Autodesk Inventor part; units mm, degrees
(part 3 of 4)
  arc A461 (22.2112, 13.7256) -> (22.0661, 14.076) centre (4.2393, 6.4866) ccw
  arc A462 (22.0661, 14.076) -> (22.3098, 14.2726) centre (18.8793, 18.2757) ccw
  arc A463 (22.3098, 14.2726) -> (22.601, 14.538) centre (18.1407, 19.1385) ccw
  arc A464 (22.601, 14.538) -> (22.939, 14.8874) centre (17.3199, 19.9858) ccw
  arc A465 (22.939, 14.8874) -> (22.7717, 15.2501) centre (4.2393, 6.4866) ccw
  arc A466 (22.7717, 15.2501) -> (22.2866, 15.22) centre (22.9993, 7.6662) ccw
  arc A467 (22.2866, 15.22) -> (21.8956, 15.171) centre (22.8881, 8.8406) ccw
  arc A468 (21.8956, 15.171) -> (21.5878, 15.1133) centre (22.7117, 9.9626) ccw
  arc A469 (21.5878, 15.1133) -> (21.4156, 15.4512) centre (4.2393, 6.4866) ccw
  arc A470 (21.4156, 15.4512) -> (21.6432, 15.6664) centre (17.9092, 19.388) ccw
  arc A471 (21.6432, 15.6664) -> (21.9127, 15.9538) centre (17.1052, 20.1902) ccw
  arc A472 (21.9127, 15.9538) -> (22.2222, 16.3286) centre (16.2205, 20.9705) ccw
  arc A473 (22.2222, 16.3286) -> (22.027, 16.6771) centre (4.2393, 6.4866) ccw
  arc A474 (22.027, 16.6771) -> (21.5457, 16.609) centre (22.8489, 9.1345) ccw
  arc A475 (21.5457, 16.609) -> (21.1598, 16.5295) centre (22.646, 10.2965) ccw
  arc A476 (21.1598, 16.5295) -> (20.8575, 16.4479) centre (22.3821, 11.4012) ccw
  arc A477 (20.8575, 16.4479) -> (20.6593, 16.7712) centre (4.2393, 6.4866) ccw
  arc A478 (20.6593, 16.7712) -> (20.8693, 17.0036) centre (16.8549, 20.4208) ccw
  arc A479 (20.8693, 17.0036) -> (21.1154, 17.3113) centre (15.9904, 21.1574) ccw
  arc A480 (21.1154, 17.3113) -> (21.3946, 17.7092) centre (15.0472, 21.8658) ccw
  arc A481 (21.3946, 17.7092) -> (21.1727, 18.0413) centre (4.2393, 6.4866) ccw
  arc A482 (21.1727, 18.0413) -> (20.6982, 17.9357) centre (22.5838, 10.5864) ccw
  arc A483 (20.6982, 17.9357) -> (20.3197, 17.8261) centre (22.2903, 11.7289) ccw
  arc A484 (20.3197, 17.8261) -> (20.0247, 17.721) centre (21.9406, 12.8095) ccw
  arc A485 (20.0247, 17.721) -> (19.8018, 18.0278) centre (4.2393, 6.4866) ccw
  arc A486 (19.8018, 18.0278) -> (19.9929, 18.2759) centre (15.7227, 21.3676) ccw
  arc A487 (19.9929, 18.2759) -> (20.2141, 18.602) centre (14.8031, 22.0342) ccw
  arc A488 (20.2141, 18.602) -> (20.4612, 19.0206) centre (13.8072, 22.6664) ccw
  arc A489 (20.4612, 19.0206) -> (20.2139, 19.3343) centre (4.2393, 6.4866) ccw
  arc A490 (20.2139, 19.3343) -> (19.7492, 19.1917) centre (22.2056, 12.0131) ccw
  arc A491 (19.7492, 19.1917) -> (19.3805, 19.0528) centre (21.8234, 13.129) ccw
  arc A492 (19.3805, 19.0528) -> (19.0946, 18.9249) centre (21.3899, 14.1788) ccw
  arc A493 (19.0946, 18.9249) -> (18.8483, 19.2133) centre (4.2393, 6.4866) ccw
  arc A494 (18.8483, 19.2133) -> (19.0194, 19.4756) centre (14.5198, 22.2227) ccw
  arc A495 (19.0194, 19.4756) -> (19.2143, 19.818) centre (13.5507, 22.8151) ccw
  arc A496 (19.2143, 19.818) -> (19.4278, 20.2547) centre (12.5083, 23.3672) ccw
  arc A497 (19.4278, 20.2547) -> (19.1566, 20.548) centre (4.2393, 6.4866) ccw
  arc A498 (19.1566, 20.548) -> (18.7045, 20.3695) centre (21.7166, 13.4056) ccw
  arc A499 (18.7045, 20.3695) -> (18.3479, 20.202) centre (21.248, 14.4882) ccw
  arc A500 (18.3479, 20.202) -> (18.0729, 20.0521) centre (20.7335, 15.5007) ccw
  arc A501 (18.0729, 20.0521) -> (17.8048, 20.3202) centre (4.2393, 6.4866) ccw
  arc A502 (17.8048, 20.3202) -> (17.9547, 20.5952) centre (13.2534, 22.9808) ccw
  arc A503 (17.9547, 20.5952) -> (18.1221, 20.9518) centre (12.2409, 23.4953) ccw
  arc A504 (18.1221, 20.9518) -> (18.3007, 21.4039) centre (11.1583, 23.964) ccw
  arc A505 (18.3007, 21.4039) -> (18.0074, 21.6751) centre (4.2393, 6.4866) ccw
  arc A506 (18.0074, 21.6751) -> (17.5707, 21.4616) centre (21.1199, 14.7556) ccw
  arc A507 (17.5707, 21.4616) -> (17.2283, 21.2667) centre (20.5678, 15.798) ccw
  arc A508 (17.2283, 21.2667) -> (16.966, 21.0956) centre (19.9754, 16.7671) ccw
  arc A509 (16.966, 21.0956) -> (16.6776, 21.3419) centre (4.2393, 6.4866) ccw
  arc A510 (16.6776, 21.3419) -> (16.8055, 21.6278) centre (11.9315, 23.6372) ccw
  arc A511 (16.8055, 21.6278) -> (16.9444, 21.9965) centre (10.8817, 24.0707) ccw
  arc A512 (16.9444, 21.9965) -> (17.087, 22.4612) centre (9.7657, 24.4529) ccw
  arc A513 (17.087, 22.4612) -> (16.7733, 22.7085) centre (4.2393, 6.4866) ccw
  arc A514 (16.7733, 22.7085) -> (16.3547, 22.4614) centre (20.4191, 16.0545) ccw
  arc A515 (16.3547, 22.4614) -> (16.0286, 22.2402) centre (19.7869, 17.0504) ccw
  arc A516 (16.0286, 22.2402) -> (15.7805, 22.0491) centre (19.1203, 17.97) ccw
  arc A517 (15.7805, 22.0491) -> (15.4737, 22.272) centre (4.2393, 6.4866) ccw
  arc A518 (15.4737, 22.272) -> (15.5788, 22.567) centre (10.5622, 24.1879) ccw
  arc A519 (15.5788, 22.567) -> (15.6884, 22.9455) centre (9.4816, 24.5376) ccw
  arc A520 (15.6884, 22.9455) -> (15.794, 23.42) centre (8.3391, 24.8311) ccw
  arc A521 (15.794, 23.42) -> (15.4619, 23.6419) centre (4.2393, 6.4866) ccw
  arc A522 (15.4619, 23.6419) -> (15.064, 23.3627) centre (19.6185, 17.2945) ccw
  arc A523 (15.064, 23.3627) -> (14.7563, 23.1166) centre (18.9101, 18.2377) ccw
  arc A524 (14.7563, 23.1166) -> (14.5239, 22.9067) centre (18.1735, 19.1022) ccw
  arc A525 (14.5239, 22.9067) -> (14.2006, 23.1048) centre (4.2393, 6.4866) ccw
  arc A526 (14.2006, 23.1048) -> (14.2822, 23.4072) centre (9.1539, 24.6294) ccw
  arc A527 (14.2822, 23.4072) -> (14.3617, 23.793) centre (8.0492, 24.8933) ccw
  arc A528 (14.3617, 23.793) -> (14.4298, 24.2743) centre (6.8872, 25.0963) ccw
  arc A529 (14.4298, 24.2743) -> (14.0813, 24.4695) centre (4.2393, 6.4866) ccw
  arc A530 (14.0813, 24.4695) -> (13.7065, 24.16) centre (18.7231, 18.4678) ccw
  arc A531 (13.7065, 24.16) -> (13.4191, 23.8905) centre (17.9429, 19.3525) ccw
  arc A532 (13.4191, 23.8905) -> (13.2039, 23.663) centre (17.1407, 20.1566) ccw
  arc A533 (13.2039, 23.663) -> (12.866, 23.8351) centre (4.2393, 6.4866) ccw
  arc A534 (12.866, 23.8351) -> (12.9236, 24.143) centre (7.7153, 24.9591) ccw
  arc A535 (12.9236, 24.143) -> (12.9727, 24.5339) centre (6.5933, 25.1355) ccw
  arc A536 (12.9727, 24.5339) -> (13.0028, 25.0191) centre (5.4189, 25.2466) ccw
  arc A537 (13.0028, 25.0191) -> (12.64, 25.1863) centre (4.2393, 6.4866) ccw
  arc A538 (12.64, 25.1863) -> (12.2907, 24.8483) centre (17.7385, 19.5672) ccw
  arc A539 (12.2907, 24.8483) -> (12.0253, 24.5571) centre (16.8912, 20.388) ccw
  arc A540 (12.0253, 24.5571) -> (11.8286, 24.3134) centre (16.0284, 21.1266) ccw
  arc A541 (11.8286, 24.3134) -> (11.4783, 24.4585) centre (4.2393, 6.4866) ccw
  arc A542 (11.4783, 24.4585) -> (11.5116, 24.7699) centre (6.2552, 25.1748) ccw
  arc A543 (11.5116, 24.7699) -> (11.5298, 25.1635) centre (5.1228, 25.2627) ccw
  arc A544 (11.5298, 25.1635) -> (11.5218, 25.6495) centre (3.9434, 25.2814) ccw
  arc A545 (11.5218, 25.6495) -> (11.147, 25.7878) centre (4.2393, 6.4866) ccw
  arc A546 (11.147, 25.7878) -> (10.8252, 25.4234) centre (16.6706, 20.5861) ccw
  arc A547 (10.8252, 25.4234) -> (10.5835, 25.1123) centre (15.7615, 21.3378) ccw
  arc A548 (10.5835, 25.1123) -> (10.4066, 24.8539) centre (14.8434, 22.0065) ccw
  arc A549 (10.4066, 24.8539) -> (10.0459, 24.9711) centre (4.2393, 6.4866) ccw
  arc A550 (10.0459, 24.9711) -> (10.0547, 25.2841) centre (4.7827, 25.2754) ccw
  arc A551 (10.0547, 25.2841) -> (10.0419, 25.6779) centre (3.647, 25.2741) ccw
  arc A552 (10.0419, 25.6779) -> (9.9958, 26.1618) centre (2.4697, 25.2002) ccw
  arc A553 (9.9958, 26.1618) -> (9.6113, 26.2702) centre (4.2393, 6.4866) ccw
  arc A554 (9.6113, 26.2702) -> (9.3192, 25.8817) centre (15.526, 21.5179) ccw
  arc A555 (9.3192, 25.8817) -> (9.1026, 25.5526) centre (14.5608, 22.1961) ccw
  arc A556 (9.1026, 25.5526) -> (8.9465, 25.2811) centre (13.5931, 22.7906) ccw
  arc A557 (8.9465, 25.2811) -> (8.5777, 25.3697) centre (4.2393, 6.4866) ccw
  arc A558 (8.5777, 25.3697) -> (8.5619, 25.6824) centre (3.3069, 25.2601) ccw
  arc A559 (8.5619, 25.6824) -> (8.5183, 26.074) centre (2.1747, 25.1697) ccw
  arc A560 (8.5183, 26.074) -> (8.4344, 26.5528) centre (1.0069, 25.0037) ccw
  arc A561 (8.4344, 26.5528) -> (8.0426, 26.6307) centre (4.2393, 6.4866) ccw
  arc A562 (8.0426, 26.6307) -> (7.7818, 26.2205) centre (14.3119, 22.3571) ccw
  arc A563 (7.7818, 26.2205) -> (7.5917, 25.8754) centre (13.2964, 22.9575) ccw
  arc A564 (7.5917, 25.8754) -> (7.4574, 25.5925) centre (12.285, 23.4742) ccw
  arc A565 (7.4574, 25.5925) -> (7.0828, 25.6518) centre (4.2393, 6.4866) ccw
  arc A566 (7.0828, 25.6518) -> (7.0425, 25.9624) centre (1.8368, 25.1291) ccw
  arc A567 (7.0425, 25.9624) -> (6.9683, 26.3493) centre (0.7152, 24.9501) ccw
  arc A568 (6.9683, 26.3493) -> (6.8471, 26.8201) centre (-0.436, 24.693) ccw
  arc A569 (6.8471, 26.8201) -> (6.4504, 26.867) centre (4.2393, 6.4866) ccw
  arc A570 (6.4504, 26.867) -> (6.2226, 26.4376) centre (13.0356, 23.0985) ccw
  arc A571 (6.2226, 26.4376) -> (6.0601, 26.0787) centre (11.9762, 23.6173) ccw
  arc A572 (6.0601, 26.0787) -> (5.9484, 25.7861) centre (10.9274, 24.0531) ccw
  arc A573 (5.9484, 25.7861) -> (5.5703, 25.8158) centre (4.2393, 6.4866) ccw
  arc A574 (5.5703, 25.8158) -> (5.5058, 26.1223) centre (0.3816, 24.8831) ccw
  arc A575 (5.5058, 26.1223) -> (5.4015, 26.5022) centre (-0.7225, 24.6167) ccw
  arc A576 (5.4015, 26.5022) -> (5.2437, 26.962) centre (-1.85, 24.27) ccw
  arc A577 (5.2437, 26.962) -> (4.8445, 26.9777) centre (4.2393, 6.4866) ccw
  arc A578 (4.8445, 26.9777) -> (4.6511, 26.5317) centre (11.7052, 23.7374) ccw
  arc A579 (4.6511, 26.5317) -> (4.5173, 26.1611) centre (10.6083, 24.1715) ccw
  arc A580 (4.5173, 26.1611) -> (4.4289, 25.8607) centre (9.5285, 24.5237) ccw
  arc A581 (4.4289, 25.8607) -> (4.0497, 25.8607) centre (4.2393, 6.4866) ccw
  arc A582 (4.0497, 25.8607) -> (3.9613, 26.1611) centre (-1.0499, 24.5237) ccw
  arc A583 (3.9613, 26.1611) -> (3.8275, 26.5317) centre (-2.1297, 24.1715) ccw
  arc A584 (3.8275, 26.5317) -> (3.6341, 26.9777) centre (-3.2265, 23.7374) ccw
  arc A585 (3.6341, 26.9777) -> (3.2349, 26.962) centre (4.2393, 6.4866) ccw
  arc A586 (3.2349, 26.962) -> (3.0771, 26.5022) centre (10.3287, 24.27) ccw
  arc A587 (3.0771, 26.5022) -> (2.9728, 26.1223) centre (9.2011, 24.6167) ccw
  arc A588 (2.9728, 26.1223) -> (2.9083, 25.8158) centre (8.097, 24.8831) ccw
  arc A589 (2.9083, 25.8158) -> (2.5302, 25.7861) centre (4.2393, 6.4866) ccw
  arc A590 (2.5302, 25.7861) -> (2.4185, 26.0787) centre (-2.4488, 24.0531) ccw
  arc A591 (2.4185, 26.0787) -> (2.2561, 26.4376) centre (-3.4976, 23.6173) ccw
  arc A592 (2.2561, 26.4376) -> (2.0283, 26.867) centre (-4.557, 23.0985) ccw
  arc A593 (2.0283, 26.867) -> (1.6316, 26.8201) centre (4.2393, 6.4866) ccw
  arc A594 (1.6316, 26.8201) -> (1.5103, 26.3493) centre (8.9146, 24.693) ccw
  arc A595 (1.5103, 26.3493) -> (1.4361, 25.9624) centre (7.7634, 24.9501) ccw
  arc A596 (1.4361, 25.9624) -> (1.3958, 25.6518) centre (6.6418, 25.1291) ccw
  arc A597 (1.3958, 25.6518) -> (1.0212, 25.5925) centre (4.2393, 6.4866) ccw
  arc A598 (1.0212, 25.5925) -> (0.887, 25.8754) centre (-3.8064, 23.4742) ccw
  arc A599 (0.887, 25.8754) -> (0.6968, 26.2205) centre (-4.8178, 22.9575) ccw
  arc A600 (0.6968, 26.2205) -> (0.436, 26.6307) centre (-5.8332, 22.3571) ccw
  arc A601 (0.436, 26.6307) -> (0.0443, 26.5528) centre (4.2393, 6.4866) ccw
  arc A602 (0.0443, 26.5528) -> (-0.0397, 26.074) centre (7.4718, 25.0037) ccw
  arc A603 (-0.0397, 26.074) -> (-0.0833, 25.6824) centre (6.3039, 25.1697) ccw
  arc A604 (-0.0833, 25.6824) -> (-0.0991, 25.3697) centre (5.1717, 25.2601) ccw
  arc A605 (-0.0991, 25.3697) -> (-0.4679, 25.2811) centre (4.2393, 6.4866) ccw
  arc A606 (-0.4679, 25.2811) -> (-0.6239, 25.5526) centre (-5.1144, 22.7906) ccw
  arc A607 (-0.6239, 25.5526) -> (-0.8405, 25.8817) centre (-6.0822, 22.1961) ccw
  arc A608 (-0.8405, 25.8817) -> (-1.1327, 26.2702) centre (-7.0474, 21.5179) ccw
  arc A609 (-1.1327, 26.2702) -> (-1.5172, 26.1618) centre (4.2393, 6.4866) ccw
  arc A610 (-1.5172, 26.1618) -> (-1.5633, 25.6779) centre (6.009, 25.2002) ccw
  arc A611 (-1.5633, 25.6779) -> (-1.576, 25.2841) centre (4.8317, 25.2741) ccw
  arc A612 (-1.576, 25.2841) -> (-1.5673, 24.9711) centre (3.6959, 25.2754) ccw
  arc A613 (-1.5673, 24.9711) -> (-1.928, 24.8539) centre (4.2393, 6.4866) ccw
  arc A614 (-1.928, 24.8539) -> (-2.1048, 25.1123) centre (-6.3648, 22.0065) ccw
  arc A615 (-2.1048, 25.1123) -> (-2.3466, 25.4234) centre (-7.2829, 21.3378) ccw
  arc A616 (-2.3466, 25.4234) -> (-2.6684, 25.7878) centre (-8.1919, 20.5861) ccw
  arc A617 (-2.6684, 25.7878) -> (-3.0431, 25.6495) centre (4.2393, 6.4866) ccw
  arc A618 (-3.0431, 25.6495) -> (-3.0512, 25.1635) centre (4.5353, 25.2814) ccw
  arc A619 (-3.0512, 25.1635) -> (-3.033, 24.7699) centre (3.3558, 25.2627) ccw
  arc A620 (-3.033, 24.7699) -> (-2.9996, 24.4585) centre (2.2234, 25.1748) ccw
  arc A621 (-2.9996, 24.4585) -> (-3.35, 24.3134) centre (4.2393, 6.4866) ccw
  arc A622 (-3.35, 24.3134) -> (-3.5466, 24.5571) centre (-7.5498, 21.1266) ccw
  arc A623 (-3.5466, 24.5571) -> (-3.8121, 24.8483) centre (-8.4126, 20.388) ccw
  arc A624 (-3.8121, 24.8483) -> (-4.1614, 25.1863) centre (-9.2598, 19.5672) ccw
  arc A625 (-4.1614, 25.1863) -> (-4.5242, 25.0191) centre (4.2393, 6.4866) ccw
  arc A626 (-4.5242, 25.0191) -> (-4.4941, 24.5339) centre (3.0597, 25.2466) ccw
  arc A627 (-4.4941, 24.5339) -> (-4.445, 24.143) centre (1.8854, 25.1355) ccw
  arc A628 (-4.445, 24.143) -> (-4.3874, 23.8351) centre (0.7634, 24.9591) ccw
  arc A629 (-4.3874, 23.8351) -> (-4.7253, 23.663) centre (4.2393, 6.4866) ccw
  arc A630 (-4.7253, 23.663) -> (-4.9404, 23.8905) centre (-8.6621, 20.1566) ccw
  arc A631 (-4.9404, 23.8905) -> (-5.2279, 24.16) centre (-9.4643, 19.3525) ccw
  arc A632 (-5.2279, 24.16) -> (-5.6027, 24.4695) centre (-10.2445, 18.4678) ccw
  arc A633 (-5.6027, 24.4695) -> (-5.9512, 24.2743) centre (4.2393, 6.4866) ccw
  arc A634 (-5.9512, 24.2743) -> (-5.8831, 23.793) centre (1.5915, 25.0963) ccw
  arc A635 (-5.8831, 23.793) -> (-5.8036, 23.4072) centre (0.4294, 24.8933) ccw
  arc A636 (-5.8036, 23.4072) -> (-5.7219, 23.1048) centre (-0.6753, 24.6294) ccw
  arc A637 (-5.7219, 23.1048) -> (-6.0453, 22.9067) centre (4.2393, 6.4866) ccw
  arc A638 (-6.0453, 22.9067) -> (-6.2776, 23.1166) centre (-9.6948, 19.1022) ccw
  arc A639 (-6.2776, 23.1166) -> (-6.5853, 23.3627) centre (-10.4315, 18.2377) ccw
  circle A640 centre (4.2393, 6.4866) radius 2
  circle A641 centre (4.2393, 6.4866) radius 18.25
  point P0 (0, 0)
  dimension "d28" = 36.5
  constraints: 1 centre point, 1 coincident
  measures "d28" diameter of A641
extrude "押し出し8" cut sketch "スケッチ2" against normal blind 0.75 contours A641
sketch "スケッチ3" plane through (0, 0, 0) normal (0, 0, -1) x (-1, 0, 0)
  arc A0 (6.9833, 23.6419) -> (6.5853, 23.3627) centre (11.1399, 17.2945) ccw
  arc A1 (6.5853, 23.3627) -> (6.2776, 23.1166) centre (10.4315, 18.2377) ccw
  arc A2 (6.2776, 23.1166) -> (6.0453, 22.9067) centre (9.6948, 19.1022) ccw
  arc A3 (6.0453, 22.9067) -> (5.7219, 23.1048) centre (-4.2393, 6.4866) ccw
  arc A4 (5.7219, 23.1048) -> (5.8036, 23.4072) centre (0.6753, 24.6294) ccw
  arc A5 (5.8036, 23.4072) -> (5.8831, 23.793) centre (-0.4294, 24.8933) ccw
  arc A6 (5.8831, 23.793) -> (5.9512, 24.2743) centre (-1.5915, 25.0963) ccw
  arc A7 (5.9512, 24.2743) -> (5.6027, 24.4695) centre (-4.2393, 6.4866) ccw
  arc A8 (5.6027, 24.4695) -> (5.2279, 24.16) centre (10.2445, 18.4678) ccw
  arc A9 (5.2279, 24.16) -> (4.9404, 23.8905) centre (9.4643, 19.3525) ccw
  arc A10 (4.9404, 23.8905) -> (4.7253, 23.663) centre (8.6621, 20.1566) ccw
  arc A11 (4.7253, 23.663) -> (4.3874, 23.8351) centre (-4.2393, 6.4866) ccw
  arc A12 (4.3874, 23.8351) -> (4.445, 24.143) centre (-0.7634, 24.9591) ccw
  arc A13 (4.445, 24.143) -> (4.4941, 24.5339) centre (-1.8854, 25.1355) ccw
  arc A14 (4.4941, 24.5339) -> (4.5242, 25.0191) centre (-3.0597, 25.2466) ccw
  arc A15 (4.5242, 25.0191) -> (4.1614, 25.1863) centre (-4.2393, 6.4866) ccw
  arc A16 (4.1614, 25.1863) -> (3.8121, 24.8483) centre (9.2598, 19.5672) ccw
  arc A17 (3.8121, 24.8483) -> (3.5466, 24.5571) centre (8.4126, 20.388) ccw
  arc A18 (3.5466, 24.5571) -> (3.35, 24.3134) centre (7.5498, 21.1266) ccw
  arc A19 (3.35, 24.3134) -> (2.9996, 24.4585) centre (-4.2393, 6.4866) ccw
  arc A20 (2.9996, 24.4585) -> (3.033, 24.7699) centre (-2.2234, 25.1748) ccw
  arc A21 (3.033, 24.7699) -> (3.0512, 25.1635) centre (-3.3558, 25.2627) ccw
  arc A22 (3.0512, 25.1635) -> (3.0431, 25.6495) centre (-4.5353, 25.2814) ccw
  arc A23 (3.0431, 25.6495) -> (2.6684, 25.7878) centre (-4.2393, 6.4866) ccw
  arc A24 (2.6684, 25.7878) -> (2.3466, 25.4234) centre (8.1919, 20.5861) ccw
  arc A25 (2.3466, 25.4234) -> (2.1048, 25.1123) centre (7.2829, 21.3378) ccw
  arc A26 (2.1048, 25.1123) -> (1.928, 24.8539) centre (6.3648, 22.0065) ccw
  arc A27 (1.928, 24.8539) -> (1.5673, 24.9711) centre (-4.2393, 6.4866) ccw
  arc A28 (1.5673, 24.9711) -> (1.576, 25.2841) centre (-3.6959, 25.2754) ccw
  arc A29 (1.576, 25.2841) -> (1.5633, 25.6779) centre (-4.8317, 25.2741) ccw
  arc A30 (1.5633, 25.6779) -> (1.5172, 26.1618) centre (-6.009, 25.2002) ccw
  arc A31 (1.5172, 26.1618) -> (1.1327, 26.2702) centre (-4.2393, 6.4866) ccw
  arc A32 (1.1327, 26.2702) -> (0.8405, 25.8817) centre (7.0474, 21.5179) ccw
  arc A33 (0.8405, 25.8817) -> (0.6239, 25.5526) centre (6.0822, 22.1961) ccw
  arc A34 (0.6239, 25.5526) -> (0.4679, 25.2811) centre (5.1144, 22.7906) ccw
  arc A35 (0.4679, 25.2811) -> (0.0991, 25.3697) centre (-4.2393, 6.4866) ccw
  arc A36 (0.0991, 25.3697) -> (0.0833, 25.6824) centre (-5.1717, 25.2601) ccw
  arc A37 (0.0833, 25.6824) -> (0.0397, 26.074) centre (-6.3039, 25.1697) ccw
  arc A38 (0.0397, 26.074) -> (-0.0443, 26.5528) centre (-7.4718, 25.0037) ccw
  arc A39 (-0.0443, 26.5528) -> (-0.436, 26.6307) centre (-4.2393, 6.4866) ccw
  arc A40 (-0.436, 26.6307) -> (-0.6968, 26.2205) centre (5.8332, 22.3571) ccw
  arc A41 (-0.6968, 26.2205) -> (-0.887, 25.8754) centre (4.8178, 22.9575) ccw
  arc A42 (-0.887, 25.8754) -> (-1.0212, 25.5925) centre (3.8064, 23.4742) ccw
  arc A43 (-1.0212, 25.5925) -> (-1.3958, 25.6518) centre (-4.2393, 6.4866) ccw
  arc A44 (-1.3958, 25.6518) -> (-1.4361, 25.9624) centre (-6.6418, 25.1291) ccw
  arc A45 (-1.4361, 25.9624) -> (-1.5103, 26.3493) centre (-7.7634, 24.9501) ccw
  arc A46 (-1.5103, 26.3493) -> (-1.6316, 26.8201) centre (-8.9146, 24.693) ccw
  arc A47 (-1.6316, 26.8201) -> (-2.0283, 26.867) centre (-4.2393, 6.4866) ccw
  arc A48 (-2.0283, 26.867) -> (-2.2561, 26.4376) centre (4.557, 23.0985) ccw
  arc A49 (-2.2561, 26.4376) -> (-2.4185, 26.0787) centre (3.4976, 23.6173) ccw
  arc A50 (-2.4185, 26.0787) -> (-2.5302, 25.7861) centre (2.4488, 24.0531) ccw
  arc A51 (-2.5302, 25.7861) -> (-2.9083, 25.8158) centre (-4.2393, 6.4866) ccw
  arc A52 (-2.9083, 25.8158) -> (-2.9728, 26.1223) centre (-8.097, 24.8831) ccw
  arc A53 (-2.9728, 26.1223) -> (-3.0771, 26.5022) centre (-9.2011, 24.6167) ccw
  arc A54 (-3.0771, 26.5022) -> (-3.2349, 26.962) centre (-10.3287, 24.27) ccw
  arc A55 (-3.2349, 26.962) -> (-3.6341, 26.9777) centre (-4.2393, 6.4866) ccw
  arc A56 (-3.6341, 26.9777) -> (-3.8275, 26.5317) centre (3.2265, 23.7374) ccw
  arc A57 (-3.8275, 26.5317) -> (-3.9613, 26.1611) centre (2.1297, 24.1715) ccw
  arc A58 (-3.9613, 26.1611) -> (-4.0497, 25.8607) centre (1.0499, 24.5237) ccw
  arc A59 (-4.0497, 25.8607) -> (-4.4289, 25.8607) centre (-4.2393, 6.4866) ccw
  arc A60 (-4.4289, 25.8607) -> (-4.5173, 26.1611) centre (-9.5285, 24.5237) ccw
  arc A61 (-4.5173, 26.1611) -> (-4.6511, 26.5317) centre (-10.6083, 24.1715) ccw
  arc A62 (-4.6511, 26.5317) -> (-4.8445, 26.9777) centre (-11.7052, 23.7374) ccw
  arc A63 (-4.8445, 26.9777) -> (-5.2437, 26.962) centre (-4.2393, 6.4866) ccw
  arc A64 (-5.2437, 26.962) -> (-5.4015, 26.5022) centre (1.85, 24.27) ccw
  arc A65 (-5.4015, 26.5022) -> (-5.5058, 26.1223) centre (0.7225, 24.6167) ccw
  arc A66 (-5.5058, 26.1223) -> (-5.5703, 25.8158) centre (-0.3816, 24.8831) ccw
  arc A67 (-5.5703, 25.8158) -> (-5.9484, 25.7861) centre (-4.2393, 6.4866) ccw
  arc A68 (-5.9484, 25.7861) -> (-6.0601, 26.0787) centre (-10.9274, 24.0531) ccw
  arc A69 (-6.0601, 26.0787) -> (-6.2226, 26.4376) centre (-11.9762, 23.6173) ccw
  arc A70 (-6.2226, 26.4376) -> (-6.4504, 26.867) centre (-13.0356, 23.0985) ccw
  arc A71 (-6.4504, 26.867) -> (-6.8471, 26.8201) centre (-4.2393, 6.4866) ccw
  arc A72 (-6.8471, 26.8201) -> (-6.9683, 26.3493) centre (0.436, 24.693) ccw
  arc A73 (-6.9683, 26.3493) -> (-7.0425, 25.9624) centre (-0.7152, 24.9501) ccw
  arc A74 (-7.0425, 25.9624) -> (-7.0828, 25.6518) centre (-1.8368, 25.1291) ccw
  arc A75 (-7.0828, 25.6518) -> (-7.4574, 25.5925) centre (-4.2393, 6.4866) ccw
  arc A76 (-7.4574, 25.5925) -> (-7.5917, 25.8754) centre (-12.285, 23.4742) ccw
  arc A77 (-7.5917, 25.8754) -> (-7.7818, 26.2205) centre (-13.2964, 22.9575) ccw
  arc A78 (-7.7818, 26.2205) -> (-8.0426, 26.6307) centre (-14.3119, 22.3571) ccw
  arc A79 (-8.0426, 26.6307) -> (-8.4344, 26.5528) centre (-4.2393, 6.4866) ccw
  arc A80 (-8.4344, 26.5528) -> (-8.5183, 26.074) centre (-1.0069, 25.0037) ccw
  arc A81 (-8.5183, 26.074) -> (-8.5619, 25.6824) centre (-2.1747, 25.1697) ccw
  arc A82 (-8.5619, 25.6824) -> (-8.5777, 25.3697) centre (-3.3069, 25.2601) ccw
  arc A83 (-8.5777, 25.3697) -> (-8.9465, 25.2811) centre (-4.2393, 6.4866) ccw
  arc A84 (-8.9465, 25.2811) -> (-9.1026, 25.5526) centre (-13.5931, 22.7906) ccw
  arc A85 (-9.1026, 25.5526) -> (-9.3192, 25.8817) centre (-14.5608, 22.1961) ccw
  arc A86 (-9.3192, 25.8817) -> (-9.6113, 26.2702) centre (-15.526, 21.5179) ccw
  arc A87 (-9.6113, 26.2702) -> (-9.9958, 26.1618) centre (-4.2393, 6.4866) ccw
  arc A88 (-9.9958, 26.1618) -> (-10.0419, 25.6779) centre (-2.4697, 25.2002) ccw
  arc A89 (-10.0419, 25.6779) -> (-10.0547, 25.2841) centre (-3.647, 25.2741) ccw
  arc A90 (-10.0547, 25.2841) -> (-10.0459, 24.9711) centre (-4.7827, 25.2754) ccw
  arc A91 (-10.0459, 24.9711) -> (-10.4066, 24.8539) centre (-4.2393, 6.4866) ccw
  arc A92 (-10.4066, 24.8539) -> (-10.5835, 25.1123) centre (-14.8434, 22.0065) ccw
  arc A93 (-10.5835, 25.1123) -> (-10.8252, 25.4234) centre (-15.7615, 21.3378) ccw
  arc A94 (-10.8252, 25.4234) -> (-11.147, 25.7878) centre (-16.6706, 20.5861) ccw
  arc A95 (-11.147, 25.7878) -> (-11.5218, 25.6495) centre (-4.2393, 6.4866) ccw
  arc A96 (-11.5218, 25.6495) -> (-11.5298, 25.1635) centre (-3.9434, 25.2814) ccw
  arc A97 (-11.5298, 25.1635) -> (-11.5116, 24.7699) centre (-5.1228, 25.2627) ccw
  arc A98 (-11.5116, 24.7699) -> (-11.4783, 24.4585) centre (-6.2552, 25.1748) ccw
  arc A99 (-11.4783, 24.4585) -> (-11.8286, 24.3134) centre (-4.2393, 6.4866) ccw
  arc A100 (-11.8286, 24.3134) -> (-12.0253, 24.5571) centre (-16.0284, 21.1266) ccw
  arc A101 (-12.0253, 24.5571) -> (-12.2907, 24.8483) centre (-16.8912, 20.388) ccw
  arc A102 (-12.2907, 24.8483) -> (-12.64, 25.1863) centre (-17.7385, 19.5672) ccw
  arc A103 (-12.64, 25.1863) -> (-13.0028, 25.0191) centre (-4.2393, 6.4866) ccw
  arc A104 (-13.0028, 25.0191) -> (-12.9727, 24.5339) centre (-5.4189, 25.2466) ccw
  arc A105 (-12.9727, 24.5339) -> (-12.9236, 24.143) centre (-6.5933, 25.1355) ccw
  arc A106 (-12.9236, 24.143) -> (-12.866, 23.8351) centre (-7.7153, 24.9591) ccw
  arc A107 (-12.866, 23.8351) -> (-13.2039, 23.663) centre (-4.2393, 6.4866) ccw
  arc A108 (-13.2039, 23.663) -> (-13.4191, 23.8905) centre (-17.1407, 20.1566) ccw
  arc A109 (-13.4191, 23.8905) -> (-13.7065, 24.16) centre (-17.9429, 19.3525) ccw
  arc A110 (-13.7065, 24.16) -> (-14.0813, 24.4695) centre (-18.7231, 18.4678) ccw
  arc A111 (-14.0813, 24.4695) -> (-14.4298, 24.2743) centre (-4.2393, 6.4866) ccw
  arc A112 (-14.4298, 24.2743) -> (-14.3617, 23.793) centre (-6.8872, 25.0963) ccw
  arc A113 (-14.3617, 23.793) -> (-14.2822, 23.4072) centre (-8.0492, 24.8933) ccw
  arc A114 (-14.2822, 23.4072) -> (-14.2006, 23.1048) centre (-9.1539, 24.6294) ccw
  arc A115 (-14.2006, 23.1048) -> (-14.5239, 22.9067) centre (-4.2393, 6.4866) ccw
  arc A116 (-14.5239, 22.9067) -> (-14.7563, 23.1166) centre (-18.1735, 19.1022) ccw
  arc A117 (-14.7563, 23.1166) -> (-15.064, 23.3627) centre (-18.9101, 18.2377) ccw
  arc A118 (-15.064, 23.3627) -> (-15.4619, 23.6419) centre (-19.6185, 17.2945) ccw
  arc A119 (-15.4619, 23.6419) -> (-15.794, 23.42) centre (-4.2393, 6.4866) ccw
  arc A120 (-15.794, 23.42) -> (-15.6884, 22.9455) centre (-8.3391, 24.8311) ccw
  arc A121 (-15.6884, 22.9455) -> (-15.5788, 22.567) centre (-9.4816, 24.5376) ccw
  arc A122 (-15.5788, 22.567) -> (-15.4737, 22.272) centre (-10.5622, 24.1879) ccw
  arc A123 (-15.4737, 22.272) -> (-15.7805, 22.0491) centre (-4.2393, 6.4866) ccw
  arc A124 (-15.7805, 22.0491) -> (-16.0286, 22.2402) centre (-19.1203, 17.97) ccw
  arc A125 (-16.0286, 22.2402) -> (-16.3547, 22.4614) centre (-19.7869, 17.0504) ccw
  arc A126 (-16.3547, 22.4614) -> (-16.7733, 22.7085) centre (-20.4191, 16.0545) ccw
  arc A127 (-16.7733, 22.7085) -> (-17.087, 22.4612) centre (-4.2393, 6.4866) ccw
  arc A128 (-17.087, 22.4612) -> (-16.9444, 21.9965) centre (-9.7657, 24.4529) ccw
  arc A129 (-16.9444, 21.9965) -> (-16.8055, 21.6278) centre (-10.8817, 24.0707) ccw
  arc A130 (-16.8055, 21.6278) -> (-16.6776, 21.3419) centre (-11.9315, 23.6372) ccw
  arc A131 (-16.6776, 21.3419) -> (-16.966, 21.0956) centre (-4.2393, 6.4866) ccw
  arc A132 (-16.966, 21.0956) -> (-17.2283, 21.2667) centre (-19.9754, 16.7671) ccw
  arc A133 (-17.2283, 21.2667) -> (-17.5707, 21.4616) centre (-20.5678, 15.798) ccw
  arc A134 (-17.5707, 21.4616) -> (-18.0074, 21.6751) centre (-21.1199, 14.7556) ccw
  arc A135 (-18.0074, 21.6751) -> (-18.3007, 21.4039) centre (-4.2393, 6.4866) ccw
  arc A136 (-18.3007, 21.4039) -> (-18.1221, 20.9518) centre (-11.1583, 23.964) ccw
  arc A137 (-18.1221, 20.9518) -> (-17.9547, 20.5952) centre (-12.2409, 23.4953) ccw
  arc A138 (-17.9547, 20.5952) -> (-17.8048, 20.3202) centre (-13.2534, 22.9808) ccw
  arc A139 (-17.8048, 20.3202) -> (-18.0729, 20.0521) centre (-4.2393, 6.4866) ccw
  arc A140 (-18.0729, 20.0521) -> (-18.3479, 20.202) centre (-20.7335, 15.5007) ccw
  arc A141 (-18.3479, 20.202) -> (-18.7045, 20.3695) centre (-21.248, 14.4882) ccw
  arc A142 (-18.7045, 20.3695) -> (-19.1566, 20.548) centre (-21.7166, 13.4056) ccw
  arc A143 (-19.1566, 20.548) -> (-19.4278, 20.2547) centre (-4.2393, 6.4866) ccw
  arc A144 (-19.4278, 20.2547) -> (-19.2143, 19.818) centre (-12.5083, 23.3672) ccw
  arc A145 (-19.2143, 19.818) -> (-19.0194, 19.4756) centre (-13.5507, 22.8151) ccw
  arc A146 (-19.0194, 19.4756) -> (-18.8483, 19.2133) centre (-14.5198, 22.2227) ccw
  arc A147 (-18.8483, 19.2133) -> (-19.0946, 18.9249) centre (-4.2393, 6.4866) ccw
  arc A148 (-19.0946, 18.9249) -> (-19.3805, 19.0528) centre (-21.3899, 14.1788) ccw
  arc A149 (-19.3805, 19.0528) -> (-19.7492, 19.1917) centre (-21.8234, 13.129) ccw
  arc A150 (-19.7492, 19.1917) -> (-20.2139, 19.3343) centre (-22.2056, 12.0131) ccw
  arc A151 (-20.2139, 19.3343) -> (-20.4612, 19.0206) centre (-4.2393, 6.4866) ccw
  arc A152 (-20.4612, 19.0206) -> (-20.2141, 18.602) centre (-13.8072, 22.6664) ccw
  arc A153 (-20.2141, 18.602) -> (-19.9929, 18.2759) centre (-14.8031, 22.0342) ccw
  arc A154 (-19.9929, 18.2759) -> (-19.8018, 18.0278) centre (-15.7227, 21.3676) ccw
  arc A155 (-19.8018, 18.0278) -> (-20.0247, 17.721) centre (-4.2393, 6.4866) ccw
  arc A156 (-20.0247, 17.721) -> (-20.3197, 17.8261) centre (-21.9406, 12.8095) ccw
  arc A157 (-20.3197, 17.8261) -> (-20.6982, 17.9357) centre (-22.2903, 11.7289) ccw
  arc A158 (-20.6982, 17.9357) -> (-21.1727, 18.0413) centre (-22.5838, 10.5864) ccw
  arc A159 (-21.1727, 18.0413) -> (-21.3946, 17.7092) centre (-4.2393, 6.4866) ccw
  arc A160 (-21.3946, 17.7092) -> (-21.1154, 17.3113) centre (-15.0472, 21.8658) ccw
  arc A161 (-21.1154, 17.3113) -> (-20.8693, 17.0036) centre (-15.9904, 21.1574) ccw
  arc A162 (-20.8693, 17.0036) -> (-20.6593, 16.7712) centre (-16.8549, 20.4208) ccw
  arc A163 (-20.6593, 16.7712) -> (-20.8575, 16.4479) centre (-4.2393, 6.4866) ccw
  arc A164 (-20.8575, 16.4479) -> (-21.1598, 16.5295) centre (-22.3821, 11.4012) ccw
  arc A165 (-21.1598, 16.5295) -> (-21.5457, 16.609) centre (-22.646, 10.2965) ccw
  arc A166 (-21.5457, 16.609) -> (-22.027, 16.6771) centre (-22.8489, 9.1345) ccw
  arc A167 (-22.027, 16.6771) -> (-22.2222, 16.3286) centre (-4.2393, 6.4866) ccw
  arc A168 (-22.2222, 16.3286) -> (-21.9127, 15.9538) centre (-16.2205, 20.9705) ccw
  arc A169 (-21.9127, 15.9538) -> (-21.6432, 15.6664) centre (-17.1052, 20.1902) ccw
  arc A170 (-21.6432, 15.6664) -> (-21.4156, 15.4512) centre (-17.9092, 19.388) ccw
  arc A171 (-21.4156, 15.4512) -> (-21.5878, 15.1133) centre (-4.2393, 6.4866) ccw
  arc A172 (-21.5878, 15.1133) -> (-21.8956, 15.171) centre (-22.7117, 9.9626) ccw
  arc A173 (-21.8956, 15.171) -> (-22.2866, 15.22) centre (-22.8881, 8.8406) ccw
  arc A174 (-22.2866, 15.22) -> (-22.7717, 15.2501) centre (-22.9993, 7.6662) ccw
  arc A175 (-22.7717, 15.2501) -> (-22.939, 14.8874) centre (-4.2393, 6.4866) ccw
  arc A176 (-22.939, 14.8874) -> (-22.601, 14.538) centre (-17.3199, 19.9858) ccw
  arc A177 (-22.601, 14.538) -> (-22.3098, 14.2726) centre (-18.1407, 19.1385) ccw
  arc A178 (-22.3098, 14.2726) -> (-22.0661, 14.076) centre (-18.8793, 18.2757) ccw
  arc A179 (-22.0661, 14.076) -> (-22.2112, 13.7256) centre (-4.2393, 6.4866) ccw
  arc A180 (-22.2112, 13.7256) -> (-22.5226, 13.7589) centre (-22.9275, 8.5025) ccw
  arc A181 (-22.5226, 13.7589) -> (-22.9161, 13.7771) centre (-23.0153, 7.3701) ccw
  arc A182 (-22.9161, 13.7771) -> (-23.4022, 13.7691) centre (-23.034, 6.1907) ccw
  arc A183 (-23.4022, 13.7691) -> (-23.5404, 13.3943) centre (-4.2393, 6.4866) ccw
  arc A184 (-23.5404, 13.3943) -> (-23.1761, 13.0725) centre (-18.3387, 18.9179) ccw
  arc A185 (-23.1761, 13.0725) -> (-22.865, 12.8308) centre (-19.0905, 18.0089) ccw
  arc A186 (-22.865, 12.8308) -> (-22.6065, 12.6539) centre (-19.7592, 17.0907) ccw
  arc A187 (-22.6065, 12.6539) -> (-22.7237, 12.2932) centre (-4.2393, 6.4866) ccw
  arc A188 (-22.7237, 12.2932) -> (-23.0368, 12.302) centre (-23.0281, 7.0301) ccw
  arc A189 (-23.0368, 12.302) -> (-23.4306, 12.2893) centre (-23.0268, 5.8943) ccw
  arc A190 (-23.4306, 12.2893) -> (-23.9145, 12.2431) centre (-22.9529, 4.717) ccw
  arc A191 (-23.9145, 12.2431) -> (-24.0229, 11.8587) centre (-4.2393, 6.4866) ccw
  arc A192 (-24.0229, 11.8587) -> (-23.6344, 11.5665) centre (-19.2706, 17.7733) ccw
  arc A193 (-23.6344, 11.5665) -> (-23.3053, 11.3499) centre (-19.9488, 16.8081) ccw
  arc A194 (-23.3053, 11.3499) -> (-23.0338, 11.1938) centre (-20.5433, 15.8404) ccw
  arc A195 (-23.0338, 11.1938) -> (-23.1223, 10.825) centre (-4.2393, 6.4866) ccw
  arc A196 (-23.1223, 10.825) -> (-23.4351, 10.8092) centre (-23.0128, 5.5542) ccw
  arc A197 (-23.4351, 10.8092) -> (-23.8267, 10.7656) centre (-22.9224, 4.422) ccw
  arc A198 (-23.8267, 10.7656) -> (-24.3055, 10.6817) centre (-22.7564, 3.2542) ccw
  arc A199 (-24.3055, 10.6817) -> (-24.3834, 10.2899) centre (-4.2393, 6.4866) ccw
  arc A200 (-24.3834, 10.2899) -> (-23.9732, 10.0291) centre (-20.1098, 16.5592) ccw
  arc A201 (-23.9732, 10.0291) -> (-23.6281, 9.839) centre (-20.7102, 15.5438) ccw
  arc A202 (-23.6281, 9.839) -> (-23.3452, 9.7047) centre (-21.2269, 14.5323) ccw
  arc A203 (-23.3452, 9.7047) -> (-23.4045, 9.3301) centre (-4.2393, 6.4866) ccw
  arc A204 (-23.4045, 9.3301) -> (-23.7151, 9.2898) centre (-22.8818, 4.0842) ccw
  arc A205 (-23.7151, 9.2898) -> (-24.102, 9.2156) centre (-22.7028, 2.9626) ccw
  arc A206 (-24.102, 9.2156) -> (-24.5728, 9.0944) centre (-22.4457, 1.8113) ccw
  arc A207 (-24.5728, 9.0944) -> (-24.6197, 8.6977) centre (-4.2393, 6.4866) ccw
  arc A208 (-24.6197, 8.6977) -> (-24.1903, 8.4699) centre (-20.8512, 15.2829) ccw
  arc A209 (-24.1903, 8.4699) -> (-23.8314, 8.3074) centre (-21.37, 14.2235) ccw
  arc A210 (-23.8314, 8.3074) -> (-23.5388, 8.1957) centre (-21.8058, 13.1747) ccw
  arc A211 (-23.5388, 8.1957) -> (-23.5685, 7.8177) centre (-4.2393, 6.4866) ccw
  arc A212 (-23.5685, 7.8177) -> (-23.875, 7.7531) centre (-22.6358, 2.6289) ccw
  arc A213 (-23.875, 7.7531) -> (-24.2549, 7.6488) centre (-22.3694, 1.5248) ccw
  arc A214 (-24.2549, 7.6488) -> (-24.7147, 7.491) centre (-22.0227, 0.3973) ccw
  arc A215 (-24.7147, 7.491) -> (-24.7304, 7.0918) centre (-4.2393, 6.4866) ccw
  arc A216 (-24.7304, 7.0918) -> (-24.2844, 6.8984) centre (-21.4901, 13.9525) ccw
  arc A217 (-24.2844, 6.8984) -> (-23.9138, 6.7646) centre (-21.9242, 12.8556) ccw
  arc A218 (-23.9138, 6.7646) -> (-23.6134, 6.6762) centre (-22.2764, 11.7758) ccw
  arc A219 (-23.6134, 6.6762) -> (-23.6134, 6.297) centre (-4.2393, 6.4866) ccw
  arc A220 (-23.6134, 6.297) -> (-23.9138, 6.2086) centre (-22.2764, 1.1974) ccw
  arc A221 (-23.9138, 6.2086) -> (-24.2844, 6.0748) centre (-21.9242, 0.1176) ccw
  arc A222 (-24.2844, 6.0748) -> (-24.7304, 5.8814) centre (-21.4901, -0.9792) ccw
  arc A223 (-24.7304, 5.8814) -> (-24.7147, 5.4823) centre (-4.2393, 6.4866) ccw
  arc A224 (-24.7147, 5.4823) -> (-24.2549, 5.3244) centre (-22.0227, 12.576) ccw
  arc A225 (-24.2549, 5.3244) -> (-23.875, 5.2201) centre (-22.3694, 11.4485) ccw
  arc A226 (-23.875, 5.2201) -> (-23.5685, 5.1556) centre (-22.6358, 10.3443) ccw
  arc A227 (-23.5685, 5.1556) -> (-23.5388, 4.7775) centre (-4.2393, 6.4866) ccw
  arc A228 (-23.5388, 4.7775) -> (-23.8314, 4.6658) centre (-21.8058, -0.2015) ccw
  arc A229 (-23.8314, 4.6658) -> (-24.1903, 4.5034) centre (-21.37, -1.2503) ccw
  arc A230 (-24.1903, 4.5034) -> (-24.6197, 4.2756) centre (-20.8512, -2.3097) ccw
  arc A231 (-24.6197, 4.2756) -> (-24.5728, 3.8789) centre (-4.2393, 6.4866) ccw
  arc A232 (-24.5728, 3.8789) -> (-24.102, 3.7576) centre (-22.4457, 11.1619) ccw
  arc A233 (-24.102, 3.7576) -> (-23.7151, 3.6834) centre (-22.7028, 10.0107) ccw
  arc A234 (-23.7151, 3.6834) -> (-23.4045, 3.6431) centre (-22.8818, 8.8891) ccw
  arc A235 (-23.4045, 3.6431) -> (-23.3452, 3.2686) centre (-4.2393, 6.4866) ccw
  arc A236 (-23.3452, 3.2686) -> (-23.6281, 3.1343) centre (-21.2269, -1.5591) ccw
  arc A237 (-23.6281, 3.1343) -> (-23.9732, 2.9442) centre (-20.7102, -2.5705) ccw
  arc A238 (-23.9732, 2.9442) -> (-24.3834, 2.6834) centre (-20.1098, -3.5859) ccw
  arc A239 (-24.3834, 2.6834) -> (-24.3055, 2.2916) centre (-4.2393, 6.4866) ccw
  arc A240 (-24.3055, 2.2916) -> (-23.8267, 2.2076) centre (-22.7564, 9.7191) ccw
  arc A241 (-23.8267, 2.2076) -> (-23.4351, 2.164) centre (-22.9224, 8.5512) ccw
  arc A242 (-23.4351, 2.164) -> (-23.1223, 2.1482) centre (-23.0128, 7.419) ccw
  arc A243 (-23.1223, 2.1482) -> (-23.0338, 1.7794) centre (-4.2393, 6.4866) ccw
  arc A244 (-23.0338, 1.7794) -> (-23.3053, 1.6234) centre (-20.5433, -2.8671) ccw
  arc A245 (-23.3053, 1.6234) -> (-23.6344, 1.4068) centre (-19.9488, -3.8349) ccw
  arc A246 (-23.6344, 1.4068) -> (-24.0229, 1.1146) centre (-19.2706, -4.8001) ccw
  arc A247 (-24.0229, 1.1146) -> (-23.9145, 0.7301) centre (-4.2393, 6.4866) ccw
  arc A248 (-23.9145, 0.7301) -> (-23.4306, 0.684) centre (-22.9529, 8.2563) ccw
  arc A249 (-23.4306, 0.684) -> (-23.0368, 0.6713) centre (-23.0268, 7.079) ccw
  arc A250 (-23.0368, 0.6713) -> (-22.7237, 0.6801) centre (-23.0281, 5.9432) ccw
  arc A251 (-22.7237, 0.6801) -> (-22.6065, 0.3194) centre (-4.2393, 6.4866) ccw
  arc A252 (-22.6065, 0.3194) -> (-22.865, 0.1425) centre (-19.7592, -4.1175) ccw
  arc A253 (-22.865, 0.1425) -> (-23.1761, -0.0993) centre (-19.0905, -5.0356) ccw
  arc A254 (-23.1761, -0.0993) -> (-23.5404, -0.4211) centre (-18.3387, -5.9446) ccw
  arc A255 (-23.5404, -0.4211) -> (-23.4022, -0.7958) centre (-4.2393, 6.4866) ccw
  arc A256 (-23.4022, -0.7958) -> (-22.9161, -0.8038) centre (-23.034, 6.7826) ccw
  arc A257 (-22.9161, -0.8038) -> (-22.5226, -0.7856) centre (-23.0153, 5.6031) ccw
  arc A258 (-22.5226, -0.7856) -> (-22.2112, -0.7523) centre (-22.9275, 4.4707) ccw
  arc A259 (-22.2112, -0.7523) -> (-22.0661, -1.1027) centre (-4.2393, 6.4866) ccw
  arc A260 (-22.0661, -1.1027) -> (-22.3098, -1.2993) centre (-18.8793, -5.3025) ccw
  arc A261 (-22.3098, -1.2993) -> (-22.601, -1.5647) centre (-18.1407, -6.1653) ccw
  arc A262 (-22.601, -1.5647) -> (-22.939, -1.9141) centre (-17.3199, -7.0125) ccw
  arc A263 (-22.939, -1.9141) -> (-22.7717, -2.2769) centre (-4.2393, 6.4866) ccw
  arc A264 (-22.7717, -2.2769) -> (-22.2866, -2.2467) centre (-22.9993, 5.307) ccw
  arc A265 (-22.2866, -2.2467) -> (-21.8956, -2.1977) centre (-22.8881, 4.1327) ccw
  arc A266 (-21.8956, -2.1977) -> (-21.5878, -2.1401) centre (-22.7117, 3.0107) ccw
  arc A267 (-21.5878, -2.1401) -> (-21.4156, -2.478) centre (-4.2393, 6.4866) ccw
  arc A268 (-21.4156, -2.478) -> (-21.6432, -2.6931) centre (-17.9092, -6.4148) ccw
  arc A269 (-21.6432, -2.6931) -> (-21.9127, -2.9806) centre (-17.1052, -7.217) ccw
  arc A270 (-21.9127, -2.9806) -> (-22.2222, -3.3554) centre (-16.2205, -7.9972) ccw
  arc A271 (-22.2222, -3.3554) -> (-22.027, -3.7039) centre (-4.2393, 6.4866) ccw
  arc A272 (-22.027, -3.7039) -> (-21.5457, -3.6358) centre (-22.8489, 3.8388) ccw
  arc A273 (-21.5457, -3.6358) -> (-21.1598, -3.5562) centre (-22.646, 2.6768) ccw
  arc A274 (-21.1598, -3.5562) -> (-20.8575, -3.4746) centre (-22.3821, 1.5721) ccw
  arc A275 (-20.8575, -3.4746) -> (-20.6593, -3.798) centre (-4.2393, 6.4866) ccw
  arc A276 (-20.6593, -3.798) -> (-20.8693, -4.0303) centre (-16.8549, -7.4475) ccw
  arc A277 (-20.8693, -4.0303) -> (-21.1154, -4.338) centre (-15.9904, -8.1842) ccw
  arc A278 (-21.1154, -4.338) -> (-21.3946, -4.736) centre (-15.0472, -8.8926) ccw
  arc A279 (-21.3946, -4.736) -> (-21.1727, -5.0681) centre (-4.2393, 6.4866) ccw
  arc A280 (-21.1727, -5.0681) -> (-20.6982, -4.9624) centre (-22.5838, 2.3868) ccw
  arc A281 (-20.6982, -4.9624) -> (-20.3197, -4.8528) centre (-22.2903, 1.2443) ccw
  arc A282 (-20.3197, -4.8528) -> (-20.0247, -4.7478) centre (-21.9406, 0.1637) ccw
  arc A283 (-20.0247, -4.7478) -> (-19.8018, -5.0546) centre (-4.2393, 6.4866) ccw
  arc A284 (-19.8018, -5.0546) -> (-19.9929, -5.3027) centre (-15.7227, -8.3944) ccw
  arc A285 (-19.9929, -5.3027) -> (-20.2141, -5.6287) centre (-14.8031, -9.0609) ccw
  arc A286 (-20.2141, -5.6287) -> (-20.4612, -6.0473) centre (-13.8072, -9.6932) ccw
  arc A287 (-20.4612, -6.0473) -> (-20.2139, -6.3611) centre (-4.2393, 6.4866) ccw
  arc A288 (-20.2139, -6.3611) -> (-19.7492, -6.2185) centre (-22.2056, 0.9602) ccw
  arc A289 (-19.7492, -6.2185) -> (-19.3805, -6.0795) centre (-21.8234, -0.1558) ccw
  arc A290 (-19.3805, -6.0795) -> (-19.0946, -5.9516) centre (-21.3899, -1.2056) ccw
  arc A291 (-19.0946, -5.9516) -> (-18.8483, -6.24) centre (-4.2393, 6.4866) ccw
  arc A292 (-18.8483, -6.24) -> (-19.0194, -6.5023) centre (-14.5198, -9.2495) ccw
  arc A293 (-19.0194, -6.5023) -> (-19.2143, -6.8447) centre (-13.5507, -9.8418) ccw
  arc A294 (-19.2143, -6.8447) -> (-19.4278, -7.2815) centre (-12.5083, -10.394) ccw
  arc A295 (-19.4278, -7.2815) -> (-19.1566, -7.5748) centre (-4.2393, 6.4866) ccw
  arc A296 (-19.1566, -7.5748) -> (-18.7045, -7.3962) centre (-21.7166, -0.4324) ccw
  arc A297 (-18.7045, -7.3962) -> (-18.3479, -7.2288) centre (-21.248, -1.5149) ccw
  arc A298 (-18.3479, -7.2288) -> (-18.0729, -7.0788) centre (-20.7335, -2.5275) ccw
  arc A299 (-18.0729, -7.0788) -> (-17.8048, -7.347) centre (-4.2393, 6.4866) ccw
  arc A300 (-17.8048, -7.347) -> (-17.9547, -7.6219) centre (-13.2534, -10.0076) ccw
  arc A301 (-17.9547, -7.6219) -> (-18.1221, -7.9786) centre (-12.2409, -10.5221) ccw
  arc A302 (-18.1221, -7.9786) -> (-18.3007, -8.4307) centre (-11.1583, -10.9907) ccw
  arc A303 (-18.3007, -8.4307) -> (-18.0074, -8.7019) centre (-4.2393, 6.4866) ccw
  arc A304 (-18.0074, -8.7019) -> (-17.5707, -8.4883) centre (-21.1199, -1.7823) ccw
  arc A305 (-17.5707, -8.4883) -> (-17.2283, -8.2934) centre (-20.5678, -2.8247) ccw
  arc A306 (-17.2283, -8.2934) -> (-16.966, -8.1224) centre (-19.9754, -3.7938) ccw
  arc A307 (-16.966, -8.1224) -> (-16.6776, -8.3687) centre (-4.2393, 6.4866) ccw
  arc A308 (-16.6776, -8.3687) -> (-16.8055, -8.6545) centre (-11.9315, -10.664) ccw
  arc A309 (-16.8055, -8.6545) -> (-16.9444, -9.0232) centre (-10.8817, -11.0974) ccw
  arc A310 (-16.9444, -9.0232) -> (-17.087, -9.488) centre (-9.7657, -11.4797) ccw
  arc A311 (-17.087, -9.488) -> (-16.7733, -9.7353) centre (-4.2393, 6.4866) ccw
  arc A312 (-16.7733, -9.7353) -> (-16.3547, -9.4881) centre (-20.4191, -3.0813) ccw
  arc A313 (-16.3547, -9.4881) -> (-16.0286, -9.267) centre (-19.7869, -4.0772) ccw
  arc A314 (-16.0286, -9.267) -> (-15.7805, -9.0759) centre (-19.1203, -4.9968) ccw
  arc A315 (-15.7805, -9.0759) -> (-15.4737, -9.2988) centre (-4.2393, 6.4866) ccw
  arc A316 (-15.4737, -9.2988) -> (-15.5788, -9.5938) centre (-10.5622, -11.2146) ccw
  arc A317 (-15.5788, -9.5938) -> (-15.6884, -9.9722) centre (-9.4816, -11.5644) ccw
  arc A318 (-15.6884, -9.9722) -> (-15.794, -10.4467) centre (-8.3391, -11.8579) ccw
  arc A319 (-15.794, -10.4467) -> (-15.4619, -10.6687) centre (-4.2393, 6.4866) ccw
  arc A320 (-15.4619, -10.6687) -> (-15.064, -10.3895) centre (-19.6185, -4.3212) ccw
  arc A321 (-15.064, -10.3895) -> (-14.7563, -10.1434) centre (-18.9101, -5.2644) ccw
  arc A322 (-14.7563, -10.1434) -> (-14.5239, -9.9334) centre (-18.1735, -6.1289) ccw
  arc A323 (-14.5239, -9.9334) -> (-14.2006, -10.1316) centre (-4.2393, 6.4866) ccw
  arc A324 (-14.2006, -10.1316) -> (-14.2822, -10.4339) centre (-9.1539, -11.6561) ccw
  arc A325 (-14.2822, -10.4339) -> (-14.3617, -10.8198) centre (-8.0492, -11.92) ccw
  arc A326 (-14.3617, -10.8198) -> (-14.4298, -11.3011) centre (-6.8872, -12.123) ccw
  arc A327 (-14.4298, -11.3011) -> (-14.0813, -11.4963) centre (-4.2393, 6.4866) ccw
  arc A328 (-14.0813, -11.4963) -> (-13.7065, -11.1867) centre (-18.7231, -5.4945) ccw
  arc A329 (-13.7065, -11.1867) -> (-13.4191, -10.9173) centre (-17.9429, -6.3793) ccw
  arc A330 (-13.4191, -10.9173) -> (-13.2039, -10.6897) centre (-17.1407, -7.1833) ccw
  arc A331 (-13.2039, -10.6897) -> (-12.866, -10.8619) centre (-4.2393, 6.4866) ccw
  arc A332 (-12.866, -10.8619) -> (-12.9236, -11.1697) centre (-7.7153, -11.9858) ccw
  arc A333 (-12.9236, -11.1697) -> (-12.9727, -11.5606) centre (-6.5933, -12.1622) ccw
  arc A334 (-12.9727, -11.5606) -> (-13.0028, -12.0458) centre (-5.4189, -12.2734) ccw
  arc A335 (-13.0028, -12.0458) -> (-12.64, -12.213) centre (-4.2393, 6.4866) ccw
  arc A336 (-12.64, -12.213) -> (-12.2907, -11.875) centre (-17.7385, -6.594) ccw
  arc A337 (-12.2907, -11.875) -> (-12.0253, -11.5839) centre (-16.8912, -7.4148) ccw
  arc A338 (-12.0253, -11.5839) -> (-11.8286, -11.3401) centre (-16.0284, -8.1534) ccw
  arc A339 (-11.8286, -11.3401) -> (-11.4783, -11.4853) centre (-4.2393, 6.4866) ccw
  arc A340 (-11.4783, -11.4853) -> (-11.5116, -11.7966) centre (-6.2552, -12.2016) ccw
  arc A341 (-11.5116, -11.7966) -> (-11.5298, -12.1902) centre (-5.1228, -12.2894) ccw
  arc A342 (-11.5298, -12.1902) -> (-11.5218, -12.6763) centre (-3.9434, -12.3081) ccw
  arc A343 (-11.5218, -12.6763) -> (-11.147, -12.8145) centre (-4.2393, 6.4866) ccw
  arc A344 (-11.147, -12.8145) -> (-10.8252, -12.4501) centre (-16.6706, -7.6128) ccw
  arc A345 (-10.8252, -12.4501) -> (-10.5835, -12.139) centre (-15.7615, -8.3646) ccw
  arc A346 (-10.5835, -12.139) -> (-10.4066, -11.8806) centre (-14.8434, -9.0332) ccw
  arc A347 (-10.4066, -11.8806) -> (-10.0459, -11.9978) centre (-4.2393, 6.4866) ccw
  arc A348 (-10.0459, -11.9978) -> (-10.0547, -12.3109) centre (-4.7827, -12.3021) ccw
  arc A349 (-10.0547, -12.3109) -> (-10.0419, -12.7046) centre (-3.647, -12.3009) ccw
  arc A350 (-10.0419, -12.7046) -> (-9.9958, -13.1886) centre (-2.4697, -12.227) ccw
  arc A351 (-9.9958, -13.1886) -> (-9.6113, -13.297) centre (-4.2393, 6.4866) ccw
  arc A352 (-9.6113, -13.297) -> (-9.3192, -12.9085) centre (-15.526, -8.5447) ccw
  arc A353 (-9.3192, -12.9085) -> (-9.1026, -12.5794) centre (-14.5608, -9.2228) ccw
  arc A354 (-9.1026, -12.5794) -> (-8.9465, -12.3079) centre (-13.5931, -9.8174) ccw
  arc A355 (-8.9465, -12.3079) -> (-8.5777, -12.3964) centre (-4.2393, 6.4866) ccw
  arc A356 (-8.5777, -12.3964) -> (-8.5619, -12.7092) centre (-3.3069, -12.2869) ccw
  arc A357 (-8.5619, -12.7092) -> (-8.5183, -13.1007) centre (-2.1747, -12.1965) ccw
  arc A358 (-8.5183, -13.1007) -> (-8.4344, -13.5796) centre (-1.0069, -12.0304) ccw
  arc A359 (-8.4344, -13.5796) -> (-8.0426, -13.6575) centre (-4.2393, 6.4866) ccw
  arc A360 (-8.0426, -13.6575) -> (-7.7818, -13.2473) centre (-14.3119, -9.3839) ccw
  arc A361 (-7.7818, -13.2473) -> (-7.5917, -12.9022) centre (-13.2964, -9.9842) ccw
  arc A362 (-7.5917, -12.9022) -> (-7.4574, -12.6193) centre (-12.285, -10.501) ccw
  arc A363 (-7.4574, -12.6193) -> (-7.0828, -12.6786) centre (-4.2393, 6.4866) ccw
  arc A364 (-7.0828, -12.6786) -> (-7.0425, -12.9891) centre (-1.8368, -12.1558) ccw
  arc A365 (-7.0425, -12.9891) -> (-6.9683, -13.3761) centre (-0.7152, -11.9769) ccw
  arc A366 (-6.9683, -13.3761) -> (-6.8471, -13.8468) centre (0.436, -11.7197) ccw
  arc A367 (-6.8471, -13.8468) -> (-6.4504, -13.8938) centre (-4.2393, 6.4866) ccw
  arc A368 (-6.4504, -13.8938) -> (-6.2226, -13.4644) centre (-13.0356, -10.1253) ccw
  arc A369 (-6.2226, -13.4644) -> (-6.0601, -13.1054) centre (-11.9762, -10.6441) ccw
  arc A370 (-6.0601, -13.1054) -> (-5.9484, -12.8128) centre (-10.9274, -11.0799) ccw
  arc A371 (-5.9484, -12.8128) -> (-5.5703, -12.8426) centre (-4.2393, 6.4866) ccw
  arc A372 (-5.5703, -12.8426) -> (-5.5058, -13.149) centre (-0.3816, -11.9099) ccw
  arc A373 (-5.5058, -13.149) -> (-5.4015, -13.529) centre (0.7225, -11.6435) ccw
  arc A374 (-5.4015, -13.529) -> (-5.2437, -13.9888) centre (1.85, -11.2968) ccw
  arc A375 (-5.2437, -13.9888) -> (-4.8445, -14.0044) centre (-4.2393, 6.4866) ccw
  arc A376 (-4.8445, -14.0044) -> (-4.6511, -13.5585) centre (-11.7052, -10.7642) ccw
  arc A377 (-4.6511, -13.5585) -> (-4.5173, -13.1879) centre (-10.6083, -11.1983) ccw
  arc A378 (-4.5173, -13.1879) -> (-4.4289, -12.8874) centre (-9.5285, -11.5505) ccw
  arc A379 (-4.4289, -12.8874) -> (-4.0497, -12.8874) centre (-4.2393, 6.4866) ccw
  arc A380 (-4.0497, -12.8874) -> (-3.9613, -13.1879) centre (1.0499, -11.5505) ccw
  arc A381 (-3.9613, -13.1879) -> (-3.8275, -13.5585) centre (2.1297, -11.1983) ccw
  arc A382 (-3.8275, -13.5585) -> (-3.6341, -14.0044) centre (3.2265, -10.7642) ccw
  arc A383 (-3.6341, -14.0044) -> (-3.2349, -13.9888) centre (-4.2393, 6.4866) ccw
  arc A384 (-3.2349, -13.9888) -> (-3.0771, -13.529) centre (-10.3287, -11.2968) ccw
  arc A385 (-3.0771, -13.529) -> (-2.9728, -13.149) centre (-9.2011, -11.6435) ccw
  arc A386 (-2.9728, -13.149) -> (-2.9083, -12.8426) centre (-8.097, -11.9099) ccw
  arc A387 (-2.9083, -12.8426) -> (-2.5302, -12.8128) centre (-4.2393, 6.4866) ccw
  arc A388 (-2.5302, -12.8128) -> (-2.4185, -13.1054) centre (2.4488, -11.0799) ccw
  arc A389 (-2.4185, -13.1054) -> (-2.2561, -13.4644) centre (3.4976, -10.6441) ccw
  arc A390 (-2.2561, -13.4644) -> (-2.0283, -13.8938) centre (4.557, -10.1253) ccw
  arc A391 (-2.0283, -13.8938) -> (-1.6316, -13.8468) centre (-4.2393, 6.4866) ccw
  arc A392 (-1.6316, -13.8468) -> (-1.5103, -13.3761) centre (-8.9146, -11.7197) ccw
  arc A393 (-1.5103, -13.3761) -> (-1.4361, -12.9891) centre (-7.7634, -11.9769) ccw
  arc A394 (-1.4361, -12.9891) -> (-1.3958, -12.6786) centre (-6.6418, -12.1558) ccw
  arc A395 (-1.3958, -12.6786) -> (-1.0212, -12.6193) centre (-4.2393, 6.4866) ccw
  arc A396 (-1.0212, -12.6193) -> (-0.887, -12.9022) centre (3.8064, -10.501) ccw
  arc A397 (-0.887, -12.9022) -> (-0.6968, -13.2473) centre (4.8178, -9.9842) ccw
  arc A398 (-0.6968, -13.2473) -> (-0.436, -13.6575) centre (5.8332, -9.3839) ccw
  arc A399 (-0.436, -13.6575) -> (-0.0443, -13.5796) centre (-4.2393, 6.4866) ccw
  arc A400 (-0.0443, -13.5796) -> (0.0397, -13.1007) centre (-7.4718, -12.0304) ccw
  arc A401 (0.0397, -13.1007) -> (0.0833, -12.7092) centre (-6.3039, -12.1965) ccw
  arc A402 (0.0833, -12.7092) -> (0.0991, -12.3964) centre (-5.1717, -12.2869) ccw
  arc A403 (0.0991, -12.3964) -> (0.4679, -12.3079) centre (-4.2393, 6.4866) ccw
  arc A404 (0.4679, -12.3079) -> (0.6239, -12.5794) centre (5.1144, -9.8174) ccw
  arc A405 (0.6239, -12.5794) -> (0.8405, -12.9085) centre (6.0822, -9.2228) ccw
  arc A406 (0.8405, -12.9085) -> (1.1327, -13.297) centre (7.0474, -8.5447) ccw
  arc A407 (1.1327, -13.297) -> (1.5172, -13.1886) centre (-4.2393, 6.4866) ccw
  arc A408 (1.5172, -13.1886) -> (1.5633, -12.7046) centre (-6.009, -12.227) ccw
  arc A409 (1.5633, -12.7046) -> (1.576, -12.3109) centre (-4.8317, -12.3009) ccw
  arc A410 (1.576, -12.3109) -> (1.5673, -11.9978) centre (-3.6959, -12.3021) ccw
  arc A411 (1.5673, -11.9978) -> (1.928, -11.8806) centre (-4.2393, 6.4866) ccw
  arc A412 (1.928, -11.8806) -> (2.1048, -12.139) centre (6.3648, -9.0332) ccw
  arc A413 (2.1048, -12.139) -> (2.3466, -12.4501) centre (7.2829, -8.3646) ccw
  arc A414 (2.3466, -12.4501) -> (2.6684, -12.8145) centre (8.1919, -7.6128) ccw
  arc A415 (2.6684, -12.8145) -> (3.0431, -12.6763) centre (-4.2393, 6.4866) ccw
  arc A416 (3.0431, -12.6763) -> (3.0512, -12.1902) centre (-4.5353, -12.3081) ccw
  arc A417 (3.0512, -12.1902) -> (3.033, -11.7966) centre (-3.3558, -12.2894) ccw
  arc A418 (3.033, -11.7966) -> (2.9996, -11.4853) centre (-2.2234, -12.2016) ccw
  arc A419 (2.9996, -11.4853) -> (3.35, -11.3401) centre (-4.2393, 6.4866) ccw
  arc A420 (3.35, -11.3401) -> (3.5466, -11.5839) centre (7.5498, -8.1534) ccw
  arc A421 (3.5466, -11.5839) -> (3.8121, -11.875) centre (8.4126, -7.4148) ccw
  arc A422 (3.8121, -11.875) -> (4.1614, -12.213) centre (9.2598, -6.594) ccw
  arc A423 (4.1614, -12.213) -> (4.5242, -12.0458) centre (-4.2393, 6.4866) ccw
  arc A424 (4.5242, -12.0458) -> (4.4941, -11.5606) centre (-3.0597, -12.2734) ccw
  arc A425 (4.4941, -11.5606) -> (4.445, -11.1697) centre (-1.8854, -12.1622) ccw
  arc A426 (4.445, -11.1697) -> (4.3874, -10.8619) centre (-0.7634, -11.9858) ccw